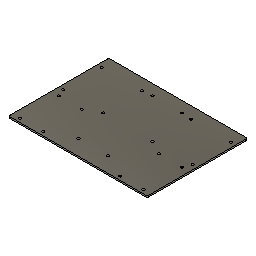
上板 v7 (Autodesk Fusion 360 design; units mm, degrees)
Autodesk Fusion 360 part; units mm, degrees
sketch "スケッチ1" plane through (0, 0, 0) normal (0, 0, 1) x (1, 0, 0)
  line L0 (0, 0) -> (180, 0)
  line L1 (180, 0) -> (180, -100)
  line L2 (180, -100) -> (0, -100)
  line L3 (0, -100) -> (0, 0)
  line L4 (0, -50) -> (180, -50) construction
  line L5 (10, -50) -> (10, -25) construction
  line L6 (10, -25) -> (40, -25) construction
  line L7 (40, -25) -> (40, -50) construction
  line L8 (90, 0) -> (90, -100) construction
  line L9 (10, -50) -> (10, -75) construction
  line L10 (10, -75) -> (40, -75) construction
  line L11 (40, -75) -> (40, -50) construction
  line L12 (140, -75) -> (140, -50) construction
  line L13 (140, -25) -> (140, -50) construction
  line L14 (170, -25) -> (140, -25) construction
  line L15 (170, -50) -> (170, -25) construction
  line L16 (170, -50) -> (170, -75) construction
  line L17 (170, -75) -> (140, -75) construction
  circle A0 centre (10, -25) radius 1.6
  circle A1 centre (40, -25) radius 1.6
  circle A2 centre (10, -75) radius 1.6
  circle A3 centre (40, -75) radius 1.6
  circle A4 centre (170, -25) radius 1.6
  circle A5 centre (140, -25) radius 1.6
  circle A6 centre (140, -75) radius 1.6
  circle A7 centre (170, -75) radius 1.6
  line L18 (40, -37.5) -> (35, -37.5)
  line L19 (35, -37.5) -> (35, -65)
  line L20 (35, -65) -> (45, -65)
  line L21 (45, -65) -> (45, -37.5)
  line L22 (45, -37.5) -> (40, -37.5)
  line L23 (145, -65) -> (135, -65)
  line L24 (135, -65) -> (135, -37.5)
  line L25 (135, -37.5) -> (140, -37.5)
  line L26 (140, -37.5) -> (145, -37.5)
  line L27 (145, -37.5) -> (145, -65)
  line L28 (90, 0) -> (64.5, 0) construction
  line L29 (64.5, 0) -> (64.5, -100) construction
  line L30 (115.5, 0) -> (115.5, -100) construction
  line L31 (64.5, -50) -> (64.5, -9) construction
  line L32 (115.5, -91) -> (115.5, -79)
  circle A8 centre (5, -95) radius 1.6
  circle A9 centre (175, -95) radius 1.6
  line L33 (0, -10) -> (180, -10)
  line L34 (180, -90) -> (0, -90)
  line L35 (0, -80) -> (180, -80)
  line L36 (0, -20) -> (180, -20)
  line L37 (0, 0) -> (180, 0)
  line L38 (180, 0) -> (180, 50)
  line L39 (180, 50) -> (0, 50)
  line L40 (0, 50) -> (0, 0)
  line L41 (90, -80) -> (90, -60)
  line L42 (90, -60) -> (109.25, -60)
  line L43 (109.25, -60) -> (70.75, -60)
  line L44 (70.75, -60) -> (70.75, 36)
  line L45 (70.75, 36) -> (109.25, 36)
  line L46 (109.25, 36) -> (109.25, -60)
  circle A10 centre (70.75, 36) radius 1.6
  circle A11 centre (109.25, 36) radius 1.6
  circle A12 centre (70.75, -60) radius 1.6
  circle A13 centre (109.25, -60) radius 1.6
  line L47 (180, 50) -> (180, 35)
  line L48 (180, 35) -> (0, 35)
  line L49 (0, 35) -> (6, 35)
  circle A14 centre (6, 35) radius 1.6
  circle A15 centre (174, 35) radius 1.6
  line L50 (6, 35) -> (58, 35)
  line L51 (58, 35) -> (58, -15)
  line L52 (58, -15) -> (6, -15)
  line L53 (6, -15) -> (6, 35)
  circle A16 centre (6, -15) radius 1.6
  circle A17 centre (58, -15) radius 1.6
  circle A18 centre (58, 35) radius 1.6
  circle A19 centre (122, 35) radius 1.6
  circle A20 centre (174, 35) radius 1.6
  circle A21 centre (174, -15) radius 1.6
  circle A22 centre (122, -15) radius 1.6
  line L54 (122, 35) -> (122, -15)
  line L55 (174, -15) -> (174, 35)
  line L56 (174, 35) -> (122, 35)
  line L57 (122, -15) -> (174, -15)
  line L58 (58, 35) -> (64, 35)
  line L59 (64, 35) -> (64, 50)
  line L60 (64, 50) -> (0, 50)
  line L61 (0, 50) -> (0, -20)
  line L62 (0, -20) -> (64, -20)
  line L63 (64, -20) -> (64, 50)
  dimension "d1" = 180
  dimension "d2" = 100
  dimension "d3" = 3.2
  dimension "d4" = 3.2
  dimension "d7" = 5
  dimension "d8" = 5
  dimension "d9" = 25.5
  dimension "d10" = 41
  dimension "d22" = 20
  dimension "d23" = 19.25
  dimension "d24" = 38.5
  dimension "d25" = 96
  dimension "d26" = 3.2
  dimension "d27" = 3.2
  dimension "d28" = 3.2
  dimension "d29" = 3.2
  dimension "d30" = 15
  dimension "d31" = 6
  dimension "d32" = 3.2
  dimension "d33" = 52
  dimension "d34" = 50
  dimension "d35" = 3.2
  dimension "d36" = 3.2
  dimension "d37" = 3.2
  dimension "d38" = 70
  constraint horizontal L0
  constraint vertical L1
  constraint horizontal L2
  constraint vertical L3
  constraint coincident L0.start L3.end
  constraint midpoint L3 L4.start
  constraint midpoint L1 L4.end
  constraint coincident L4 L5.start
  constraint perpendicular L4 L5
  constraint perpendicular L3 L6
  constraint coincident L4 L7.end
  constraint perpendicular L4 L7
  constraint midpoint L0 L8.start
  constraint midpoint L2 L8.end
  constraint symmetric L4 L5.start L9.start
  constraint symmetric L4 L5.end L9.end
  constraint symmetric L4 L6.end L10.end
  constraint symmetric L4 L7.end L11.end
  constraint symmetric L5.start L8 L15.start
  constraint symmetric L5.end L8 L14.start
  constraint symmetric L6.end L8 L13.start
  constraint symmetric L7.end L8 L12.end
  constraint symmetric L8 L5.start L15.start
  constraint symmetric L8 L9.end L16.end
  constraint symmetric L8 L10.end L12.start
  constraint symmetric L8 L7.end L12.end
  constraint coincident L5.end L6.start
  constraint coincident L6.end L7.start
  constraint symmetric L4 A0 A2
  constraint symmetric L4 A1 A3
  constraint symmetric L8 A0 A4
  constraint symmetric L8 A1 A5
  constraint symmetric L8 A2 A7
  constraint symmetric L8 A3 A6
  constraint midpoint L7 L18.start
  constraint perpendicular L7 L18
  constraint perpendicular L4 L19
  constraint perpendicular L11 L20
  constraint perpendicular L20 L21
  constraint perpendicular L7 L22
  constraint symmetric L8 L18.start L25.end
  constraint symmetric L8 L18.end L26.end
  constraint symmetric L8 L19.end L23.start
  constraint symmetric L8 L20.end L23.end
  constraint symmetric L8 L21.end L24.end
  constraint perpendicular L8 L28
  constraint coincident L2 L29.end
  constraint perpendicular L2 L29
  constraint symmetric L8 L28.end L30.start
  constraint symmetric L8 L29.end L30.end
  constraint midpoint L29 L31.start
  constraint perpendicular L4 L31
  constraint coincident L3 L33.start
  constraint coincident L1 L33.end
  constraint perpendicular L1 L33
  constraint coincident L1 L34.start
  constraint coincident L3 L34.end
  constraint perpendicular L3 L34
  constraint coincident L3 L35.start
  constraint coincident L1 L35.end
  constraint perpendicular L1 L35
  constraint coincident L3 L36.start
  constraint coincident L1 L36.end
  constraint perpendicular L1 L36
  constraint horizontal L37
  constraint vertical L38
  constraint horizontal L39
  constraint vertical L40
  constraint midpoint L35 L41.start
  constraint perpendicular L35 L41
  constraint perpendicular L41 L42
  constraint horizontal L43
  constraint vertical L44
  constraint horizontal L45
  constraint vertical L46
  constraint coincident L44.end L45.start
  constraint coincident L45.end L46.start
  constraint coincident L43.end L44.start
  constraint coincident L42.end L43.start
  constraint perpendicular L39 L47
  constraint coincident L40 L48.end
  constraint perpendicular L40 L48
  constraint perpendicular L40 L49
  constraint coincident L49.end A14.centre
  constraint symmetric L8 A14 A15
  constraint horizontal L50
  constraint vertical L51
  constraint horizontal L52
  constraint vertical L53
  constraint coincident L52.end L53.start
  constraint coincident L51.end L52.start
  constraint coincident L50.end L51.start
  constraint symmetric L8 A14 A20
  constraint symmetric L8 L49.end A15.centre
  constraint symmetric L8 L50.end A19.centre
  constraint symmetric L8 L51.end A22.centre
  constraint symmetric L8 L52.end A21.centre
  constraint symmetric L8 A16 A21
  constraint symmetric L8 A17 A22
  constraint symmetric L8 A18 A19
  constraint coincident L48 L58.end
  constraint coincident L39 L59.end
  constraint perpendicular L39 L59
  constraint horizontal L60
  constraint vertical L61
  constraint horizontal L62
  constraint vertical L63
  measures "d1" distance of L0.start L0.end
  measures "d2" distance of L0.start L2.end
  measures "d3" diameter of A0
  measures "d4" diameter of A1
  measures "d7" distance of L18.start L18.end
  measures "d8" distance of L18.start L21.end
  measures "d9" distance of L8.start L28.end
  measures "d10" distance of L31.start L31.end
  measures "d22" distance of L41.start L41.end
  measures "d23" distance of L41.end L42.end
  measures "d24" distance of L42.end L43.end
  measures "d25" distance of L42.end L45.end
  measures "d26" diameter of A10
  measures "d27" diameter of A11
  measures "d28" diameter of A12
  measures "d29" diameter of A13
  measures "d30" distance of L38.end L47.end
  measures "d31" distance of L48.end L49.end
  measures "d32" diameter of A14
  measures "d33" distance of L49.end L50.end
  measures "d34" distance of L49.end L52.end
  measures "d35" diameter of A16
  measures "d36" diameter of A17
  measures "d37" diameter of A18
  measures "d38" distance of L59.end L62.end
extrude "押し出し1" add sketch "スケッチ1" along normal blind 2 contours L0 L37 L40 L48 L49 A14 L53 L61 | L0 L3 L33 L37 L53 L61 | L0 L37 L48 A14 L50 L51 L53 A18 | L0 L33 L37 L51 L53 | L3 L33 L36 L51 L52 L53 A16 A17 L61 L62 L63 | L39 L40 L48 L49 A14 L50 A18 L58 L59 L60 L61 L63 | L0 L37 L48 L51 A18 L58 L63 | L0 L33 L37 L51 L63 | L33 L51 L52 L53 A16 A17 | L3 L35 L36 L41 L43 L44 A12 L62 | L0 L37 L44 A10 L48 L63 | L0 L33 L37 L44 L63 | L33 L36 L44 L63 | L38 L39 L45 A10 A11 L47 L48 A15 A19 A20 L56 L59 L63 | L0 L37 L44 L46 A10 A11 L48 | L0 L33 L37 L44 L46 | L1 L35 L36 L41 L42 L43 L46 A13 | L33 L36 L44 L46 | L36 L42 L43 L44 L46 A12 A13 | L0 L37 L46 A11 L48 A19 L54 | L0 L33 L37 L46 L54 | L1 L33 L36 L46 A21 A22 L54 L55 L57 | L0 L37 L38 L48 A15 A20 L55 | L0 L37 L48 A15 A19 A20 L54 L55 L56 | L0 L33 L37 L54 L55 | L45 A10 A11 L48 | L0 L1 L33 L37 L55 | L33 A21 A22 L54 L55 L57 | L18 L19 L20 L21 L22 | L23 L24 L25 L26 L27
fillet "フィレット1" radius 2 4 edges at (0, -80, 1) (180, -80, 1) (0, 50, 1) (180, 50, 1)
equation "d9 = ( 51 / 2 ) * 1 mm"
equation "d10 = ( 82 / 2 ) * 1 mm"
